Autodesk Inventor part; units mm, degrees
(part 2 of 2)
  point P158 (41.6667, -16.6667)
  point P159 (50, -8.3333)
  point P160 (66.6667, -16.6667)
  point P161 (58.3333, -16.6667)
  point P162 (66.6667, -8.3333)
  point P163 (83.3333, -16.6667)
  point P164 (75, -16.6667)
  point P165 (83.3333, -8.3333)
  point P166 (-83.3333, 0)
  point P167 (-91.6667, 0)
  point P168 (-83.3333, 8.3333)
  point P169 (-66.6667, 0)
  point P170 (-75, 0)
  point P171 (-66.6667, 8.3333)
  point P172 (-50, 0)
  point P173 (-58.3333, 0)
  point P174 (-50, 8.3333)
  point P175 (-33.3333, 0)
  point P176 (-41.6667, 0)
  point P177 (-33.3333, 8.3333)
  point P178 (-16.6667, 0)
  point P179 (-25, 0)
  point P180 (-16.6667, 8.3333)
  point P181 (0, 0)
  point P182 (-8.3333, 0)
  point P183 (0, 8.3333)
  point P184 (16.6667, 0)
  point P185 (8.3333, 0)
  point P186 (16.6667, 8.3333)
  point P187 (33.3333, 0)
  point P188 (25, 0)
  point P189 (33.3333, 8.3333)
  point P190 (50, 0)
  point P191 (41.6667, 0)
  point P192 (50, 8.3333)
  point P193 (66.6667, 0)
  point P194 (58.3333, 0)
  point P195 (66.6667, 8.3333)
  point P196 (83.3333, 0)
  point P197 (75, 0)
  point P198 (83.3333, 8.3333)
  point P199 (-83.3333, 16.6667)
  dimension "d108" = 16.6667
  dimension "d109" = 16.6667
  dimension "gridOCell_XOffset" = 91.6667
  dimension "gridOCell_YOffset" = 91.6667
  dimension "d115" = 16.6667
  dimension "d118" = 16.6667
  constraints: 968 end point, 2 collinear, 2 horizontal, 2 midpoint, 2 parallel, 1 horizontal alignment, 1 perpendicular, 1 vertical, 1 vertical alignment, 1318 other
  measures "d108" distance of L84.end L85.end
  measures "d109" distance of L85.end L86.end
  measures "gridOCell_XOffset" horizontal distance of L86.end point (0, 0)
  measures "gridOCell_YOffset" horizontal distance of L86.end point (0, 0)
  measures "d115" distance of L84.start L88.start
  measures "d118" distance of L84.start L128.start
sketch "Sketch15" plane through (0, 0, 1.5) normal (0, 0, 1) x (1, 0, 0)
  line L0 (88, 108) -> (108, 108) projected
  line L1 (88, 105) -> (88, 108) projected
  line L2 (88, 105) -> (68.8, 105) projected
  line L3 (68.8, 108) -> (68.8, 105) projected
  line L4 (48.8, 108) -> (68.8, 108) projected
  line L5 (48.8, 105) -> (48.8, 108) projected
  line L6 (48.8, 105) -> (29.6, 105) projected
  line L7 (29.6, 108) -> (29.6, 105) projected
  line L8 (9.6, 108) -> (29.6, 108) projected
  line L9 (9.6, 105) -> (9.6, 108) projected
  line L10 (9.6, 105) -> (-9.6, 105) projected
  line L11 (-9.6, 108) -> (-9.6, 105) projected
  line L12 (-29.6, 108) -> (-9.6, 108) projected
  line L13 (-29.6, 105) -> (-29.6, 108) projected
  line L14 (-29.6, 105) -> (-48.8, 105) projected
  line L15 (-48.8, 108) -> (-48.8, 105) projected
  line L16 (-68.8, 108) -> (-48.8, 108) projected
  line L17 (-68.8, 105) -> (-68.8, 108) projected
  line L18 (-68.8, 105) -> (-88, 105) projected
  line L19 (-88, 108) -> (-88, 105) projected
  line L20 (-108, 108) -> (-88, 108) projected
  line L21 (-108, 108) -> (-108, 88) projected
  line L22 (-108, 88) -> (-105, 88) projected
  line L23 (-105, 88) -> (-105, 68.8) projected
  line L24 (-105, 68.8) -> (-108, 68.8) projected
  line L25 (-108, 68.8) -> (-108, 48.8) projected
  line L26 (-108, 48.8) -> (-105, 48.8) projected
  line L27 (-105, 48.8) -> (-105, 29.6) projected
  line L28 (-105, 29.6) -> (-108, 29.6) projected
  line L29 (-108, 29.6) -> (-108, 9.6) projected
  line L30 (-108, 9.6) -> (-105, 9.6) projected
  line L31 (-105, 9.6) -> (-105, -9.6) projected
  line L32 (-105, -9.6) -> (-108, -9.6) projected
  line L33 (-108, -9.6) -> (-108, -29.6) projected
  line L34 (-108, -29.6) -> (-105, -29.6) projected
  line L35 (-105, -29.6) -> (-105, -48.8) projected
  line L36 (-105, -48.8) -> (-108, -48.8) projected
  line L37 (-108, -48.8) -> (-108, -68.8) projected
  line L38 (-108, -68.8) -> (-105, -68.8) projected
  line L39 (-105, -68.8) -> (-105, -88) projected
  line L40 (-105, -88) -> (-108, -88) projected
  line L41 (-108, -88) -> (-108, -108) projected
  line L42 (-108, -108) -> (-88, -108) projected
  line L43 (-88, -108) -> (-88, -105) projected
  line L44 (-88, -105) -> (-68.8, -105) projected
  line L45 (-68.8, -105) -> (-68.8, -108) projected
  line L46 (-68.8, -108) -> (-48.8, -108) projected
  line L47 (-48.8, -108) -> (-48.8, -105) projected
  line L48 (-48.8, -105) -> (-29.6, -105) projected
  line L49 (-29.6, -105) -> (-29.6, -108) projected
  line L50 (-29.6, -108) -> (-9.6, -108) projected
  line L51 (-9.6, -108) -> (-9.6, -105) projected
  line L52 (-9.6, -105) -> (9.6, -105) projected
  line L53 (9.6, -105) -> (9.6, -108) projected
  line L54 (9.6, -108) -> (29.6, -108) projected
  line L55 (29.6, -108) -> (29.6, -105) projected
  line L56 (29.6, -105) -> (48.8, -105) projected
  line L57 (48.8, -105) -> (48.8, -108) projected
  line L58 (48.8, -108) -> (68.8, -108) projected
  line L59 (68.8, -108) -> (68.8, -105) projected
  line L60 (68.8, -105) -> (88, -105) projected
  line L61 (88, -105) -> (88, -108) projected
  line L62 (88, -108) -> (108, -108) projected
  line L63 (108, -108) -> (108, -88) projected
  line L64 (105, -88) -> (108, -88) projected
  line L65 (105, -88) -> (105, -68.8) projected
  line L66 (108, -68.8) -> (105, -68.8) projected
  line L67 (108, -48.8) -> (108, -68.8) projected
  line L68 (105, -48.8) -> (108, -48.8) projected
  line L69 (105, -48.8) -> (105, -29.6) projected
  line L70 (108, -29.6) -> (105, -29.6) projected
  line L71 (108, -9.6) -> (108, -29.6) projected
  line L72 (105, -9.6) -> (108, -9.6) projected
  line L73 (105, -9.6) -> (105, 9.6) projected
  line L74 (108, 9.6) -> (105, 9.6) projected
  line L75 (108, 29.6) -> (108, 9.6) projected
  line L76 (105, 29.6) -> (108, 29.6) projected
  line L77 (105, 29.6) -> (105, 48.8) projected
  line L78 (108, 48.8) -> (105, 48.8) projected
  line L79 (108, 68.8) -> (108, 48.8) projected
  line L80 (105, 68.8) -> (108, 68.8) projected
  line L81 (105, 68.8) -> (105, 88) projected
  line L82 (108, 88) -> (105, 88) projected
  line L83 (108, 108) -> (108, 88) projected
  line L84 (-87, 109) -> (-87, 104)
  line L85 (-87, 104) -> (-69.8, 104)
  line L86 (-69.8, 104) -> (-69.8, 109)
  line L87 (-69.8, 109) -> (-47.8, 109)
  line L88 (-47.8, 109) -> (-47.8, 104)
  line L89 (-47.8, 104) -> (-30.6, 104)
  line L90 (-30.6, 104) -> (-30.6, 109)
  line L91 (-30.6, 109) -> (-8.6, 109)
  line L92 (-8.6, 109) -> (-8.6, 104)
  line L93 (-8.6, 104) -> (8.6, 104)
  line L94 (8.6, 104) -> (8.6, 109)
  line L95 (8.6, 109) -> (30.6, 109)
  line L96 (30.6, 109) -> (30.6, 104)
  line L97 (30.6, 104) -> (47.8, 104)
  line L98 (47.8, 104) -> (47.8, 109)
  line L99 (47.8, 109) -> (69.8, 109)
  line L100 (69.8, 109) -> (69.8, 104)
  line L101 (69.8, 104) -> (87, 104)
  line L102 (87, 104) -> (87, 109)
  line L103 (87, 109) -> (109, 109)
  line L104 (109, 109) -> (109, 87)
  line L105 (109, 87) -> (104, 87)
  line L106 (104, 87) -> (104, 69.8)
  line L107 (104, 69.8) -> (109, 69.8)
  line L108 (109, 69.8) -> (109, 47.8)
  line L109 (109, 47.8) -> (104, 47.8)
  line L110 (104, 47.8) -> (104, 30.6)
  line L111 (104, 30.6) -> (109, 30.6)
  line L112 (109, 30.6) -> (109, 8.6)
  line L113 (109, 8.6) -> (104, 8.6)
  line L114 (104, 8.6) -> (104, -8.6)
  line L115 (104, -8.6) -> (109, -8.6)
  line L116 (109, -8.6) -> (109, -30.6)
  line L117 (109, -30.6) -> (104, -30.6)
  line L118 (104, -30.6) -> (104, -47.8)
  line L119 (104, -47.8) -> (109, -47.8)
  line L120 (109, -47.8) -> (109, -69.8)
  line L121 (109, -69.8) -> (104, -69.8)
  line L122 (104, -69.8) -> (104, -87)
  line L123 (104, -87) -> (109, -87)
  line L124 (109, -87) -> (109, -109)
  line L125 (109, -109) -> (87, -109)
  line L126 (87, -109) -> (87, -104)
  line L127 (87, -104) -> (69.8, -104)
  line L128 (69.8, -104) -> (69.8, -109)
  line L129 (69.8, -109) -> (47.8, -109)
  line L130 (47.8, -109) -> (47.8, -104)
  line L131 (47.8, -104) -> (30.6, -104)
  line L132 (30.6, -104) -> (30.6, -109)
  line L133 (30.6, -109) -> (8.6, -109)
  line L134 (8.6, -109) -> (8.6, -104)
  line L135 (8.6, -104) -> (-8.6, -104)
  line L136 (-8.6, -104) -> (-8.6, -109)
  line L137 (-8.6, -109) -> (-30.6, -109)
  line L138 (-30.6, -109) -> (-30.6, -104)
  line L139 (-30.6, -104) -> (-47.8, -104)
  line L140 (-47.8, -104) -> (-47.8, -109)
  line L141 (-47.8, -109) -> (-69.8, -109)
  line L142 (-69.8, -109) -> (-69.8, -104)
  line L143 (-69.8, -104) -> (-87, -104)
  line L144 (-87, -104) -> (-87, -109)
  line L145 (-87, -109) -> (-109, -109)
  line L146 (-109, -109) -> (-109, -87)
  line L147 (-109, -87) -> (-104, -87)
  line L148 (-104, -87) -> (-104, -69.8)
  line L149 (-104, -69.8) -> (-109, -69.8)
  line L150 (-109, -69.8) -> (-109, -47.8)
  line L151 (-109, -47.8) -> (-104, -47.8)
  line L152 (-104, -47.8) -> (-104, -30.6)
  line L153 (-104, -30.6) -> (-109, -30.6)
  line L154 (-109, -30.6) -> (-109, -8.6)
  line L155 (-109, -8.6) -> (-104, -8.6)
  line L156 (-104, -8.6) -> (-104, 8.6)
  line L157 (-104, 8.6) -> (-109, 8.6)
  line L158 (-109, 8.6) -> (-109, 30.6)
  line L159 (-109, 30.6) -> (-104, 30.6)
  line L160 (-104, 30.6) -> (-104, 47.8)
  line L161 (-104, 47.8) -> (-109, 47.8)
  line L162 (-109, 47.8) -> (-109, 69.8)
  line L163 (-109, 69.8) -> (-104, 69.8)
  line L164 (-104, 69.8) -> (-104, 87)
  line L165 (-104, 87) -> (-109, 87)
  line L166 (-109, 87) -> (-109, 109)
  line L167 (-109, 109) -> (-87, 109)
  point P0 (0, 0)
  dimension "d70" = 1
  constraints: 168 end point, 83 other
  measures "d70" distance between parallel lines of L20 L167
ref_plane "Work Plane3" through (0, 0, 0) normal (0, 1, 0) x (-1, 0, 0)
equation "\"FrontFaceBaseWidth\" = ClockWidth - 2 * FrontFaceTabDepth"
equation "\"FrontFaceBaseHeight\" = ClockHeight - 2 * FrontFaceTabDepth"
equation "\"FrontFaceThickness\" = Ply3mm"
equation "\"d6\" = TabDepth"
equation "\"FrontFaceTabWidth\" = TabWidth"
equation "\"d8\" = FrontFaceTabDepth"
equation "\"d9\" = FrontFaceThickness"
equation "\"d14\" = FrontFaceTabDepth"
equation "\"d15\" = FrontFaceTabDepth"
equation "\"d16\" = FrontFaceTabWidth"
equation "\"d17\" = FrontFaceThickness"
equation "\"d68\" = ClockWidth"
equation "\"d69\" = ClockDepth"
equation "\"TopFaceThickness\" = Ply3mm"
equation "\"d25\" = FrontFaceTabWidth"
equation "\"TopFaceFrontSlotDepth\" = FrontFaceThickness"
equation "\"d27\" = TopFaceThickness"
equation "\"d33\" = TabDepth"
equation "\"d34\" = TopFaceThickness"
equation "\"d38\" = FrontFaceTopTabSpacing"
equation "\"TabDepth\" = Ply3mm"
equation "\"SideFaceBaseHeight\" = ClockHeight - 2 * FrontFaceThickness"
equation "\"SideFaceBaseDepth\" = ClockDepth"
equation "\"SideFaceThickness\" = Ply3mm"
equation "\"SideFaceTabWidth\" = TopSideSlotWidth"
equation "\"SideTopTabDepth\" = TopFaceThickness"
equation "\"d56\" = SideFaceThickness"
equation "\"d60\" = TopFaceSlotsSideSpcaing"
equation "\"d61\" = FrontFaceThickness"
equation "\"d62\" = FrontFaceTabWidth"
equation "\"d63\" = SideFaceThickness"
equation "\"d67\" = FrontFaceSideTabSpacing"
equation "\"d76\" = FrontFaceBaseHeight"
equation "\"d77\" = FrontFaceBaseWidth"
equation "\"MiddleThickness\" = Ply3mm"
equation "\"d80\" = SideFaceThickness"
equation "\"MiddleTabWidth\" = TabWidth"
equation "\"d82\" = Ply3mm"
equation "\"d86\" = MiddleSideTabSpacing"
equation "\"d87\" = TopFaceThickness"
equation "\"MiddleBottomTabWidth\" = MiddleTabWidth"
equation "\"d89\" = MiddleThickness"
equation "\"d93\" = MiddleBottomTabSpacing"
equation "\"d94\" = TopFaceThickness"
equation "\"d95\" = MiddleBottomTabWidth"
equation "\"d96\" = MiddleThickness"
equation "\"d100\" = MiddleBottomTabSpacing"
equation "\"d101\" = SideFaceThickness"
equation "\"d102\" = MiddleTabWidth"
equation "\"d103\" = MiddleThickness"
equation "\"d70\" = kerf"
equation "\"FrontFaceTabDepth\" = TabDepth"
equation "\"ClockHeight\" = 216"
equation "\"ClockWidth\" = 216"
equation "\"ClockDepth\" = 60"
equation "\"Ply3mm\" = 3"
equation "\"TabWidth\" = 20"
equation "\"kerf\" = 1"
equation "\"MiddleFrontSeparation\" = 17"
equation "\"MiddleSideTabSpacing\" = 2 * MiddleTabWidth"
equation "\"MiddleBottomTabSpacing\" = MiddleSideTabSpacing"
equation "\"gridCellHeight\" = 16.66667"
equation "\"gridCellWidth\" = 16.66667"
equation "\"FrontFaceTopTabSpacing\" = 39.2"
equation "\"TopFaceSlotsSideSpcaing\" = 40"
equation "\"FrontFaceSideTabSpacing\" = 39.2"
